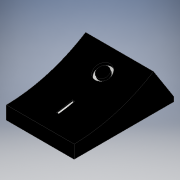
# Autodesk Inventor part: CWSB2-nonillumin_rocker
Saved by Autodesk Inventor 2019 (Build 230136000, 136)
## iProperties
Created: 2024-03-12
Part Number: CWSB2-nonillumin_rocker
Material: Generic
Catalog Web Link: www.cadenas.de
Description: CWSB - Miniature Power Rockers -nonillumin_rocker-
Vendor: NKKSWITCHES
Document SubType Name: Modeling
Designer: psAdmin
Manufacturer: NKKSWITCHES
Mass: 0.533919 g
Surface Area: 5.033 cm^2
Volume: 0.533919 cm^3
Density: 1 g/cm^3
Appearance: PSOLRGB-0-0-0
Category: PARTsolutions
Company: NKKSWITCHES
Title: CWSB2-nonillumin_rocker
Author: Cadenas PARTsolutions
PSOL_IDENT_0: {$CADENAS_DATA/23d-libs/nkkswitches/rocker/cw_nonillumin/parts/cwsb_nonillumin_rocker.prj},234 {VTYP=
PSOL_IDENT_1: 3D},{NB=CWSB2-nonillumin_rocker},{LINA=CWSB2-nonillumin_rocker},{NN=CWSB - Miniature Power Rockers -
PSOL_IDENT_2: nonillumin_rocker},{DATE=09.02.2024 16:13:46},{GEOMDATE=27.05.2013 08:55:00},{VERSION=},{LINEID=10},
PSOL_IDENT_3: {WBVAR=INSCR},{WBNUMERIC=}  {NB=CWSB2-nonillumin_rocker},{LINA=CWSB2-nonillumin_rocker},{KT=DUMMY},{
PSOL_IDENT_4: PN=CWSB2},{SRS=CWSB},{INSCR=2}
NB: CWSB2-nonillumin_rocker
NN: CWSB - Miniature Power Rockers -nonillumin_rocker
NBSYN: $PN.-nonillumin_rocker
LINA: CWSB2-nonillumin_rocker
CATALOG: NKK Switches
PN: CWSB2
SRS: CWSB
INSCR: 2 - Vertical
SUPPLIER: NKKSWITCHES
ARTICLENO: CWSB2-nonillumin_rocker
BOMINFO: CWSB2-nonillumin_rocker
CREATOR: CADENAS GmbH
Autodesk Inventor part; units mm, degrees
sketch "Sketch_2" plane through (0, 0, 0) normal (1, 0, 0) x (0, 1, 0)
  line L0 (2.0701, 7.7724) -> (0, 7.7724)
  line L1 (0, 7.7724) -> (0, -7.7724)
  line L2 (0, -7.7724) -> (0.7455, -7.7724)
  line L3 (0.7455, -7.7724) -> (5.6896, -4.6127)
  arc A0 (2.0701, 7.7724) -> (5.6896, -4.6127) centre (25.9234, 8.0219) ccw
  constraints: 8 end point, 2 point on circle, 1 centre point
extrude "Extrusion1" add sketch "Sketch_2" along normal mid plane 10.5918
sketch "Sketch_3" plane through (0, 3.2333, 0.3287) normal (0, 0.9239, 0.3827) x (1, 0, 0)
  circle A0 centre (0, 2.54) radius 1.27
  circle A1 centre (0, 2.54) radius 0.889
  constraints: 2 centre point
extrude "Extrusion2" cut sketch "Sketch_3" along normal mid plane 0.762
sketch "Sketch_4" plane through (0, 3.2333, 0.3287) normal (0, 0.9877, 0.1564) x (1, 0, 0)
  line L0 (-0.1905, -4.826) -> (0.1905, -4.826)
  line L1 (0.1905, -4.826) -> (0.1905, -2.286)
  line L2 (0.1905, -2.286) -> (-0.1905, -2.286)
  line L3 (-0.1905, -2.286) -> (-0.1905, -4.826)
  constraints: 8 end point
extrude "Extrusion3" cut sketch "Sketch_4" along normal mid plane 0.762
ref_plane "to_body_XY" through (0, 0, 0) normal (0, 1, 0) x (1, 0, 0)
ref_plane "to_body_YZ" through (0, 0, 0) normal (1, 0, 0) x (0, 0, -1)
ref_plane "to_body_ZX" through (0, 0, 0) normal (0, 0, -1) x (0, 1, 0)
body "Solid1"
